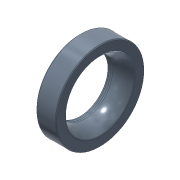
# Autodesk Inventor part: NA-45-h-Crown-129
Saved by Autodesk Inventor 2020.2 (Build 242310000, 310)
## iProperties
Created: 2020-09-21
Part Number: NA-45-h-Crown-129
Material: 19 436.4
Description: STAHOVACI KROUZEK
Document SubType Name: Modeling
Designer: Jurek
Density: 7.85 g/cm^3
Appearance: Ocelově modrá
Mass: 172.989 g
Surface Area: 71.9063 cm^2
Volume: 22.0368 cm^3
User Status: Rozpracováno
Category: B
Hmotnost (kg): 0,17
Rozmer_A: 60
Rozmer_B: 0
Rozmer_C: 0
Rozmer_D: 14
Rada vyrobku: 4100
Prumer nadobky: 45
Cislo artiklu: 4451101286
C. variantniho vykresu: NA-45-h-Crown-127
Jednotka: ks
Cisty rozmer: =Ø<Rozmer_A> - <Rozmer_D>
Predpona: Ø
Stroj na lince: Stahovací lis
RAZ Poznamka 1: ISO 2768-mH
RAZ Poznamka 2: NEOZNAČENÉ HRANY OJEHLIT
RAZ Poznamka 3: KALIT NA 58 - 60 HRc
DXF: Ne
QAD_code: M
Rizeni davek: L
Author: Správce
Revision Number: 00
Autodesk Inventor part; units mm, degrees
ref_plane "YZ Plane" through (0, 0, 0) normal (1, 0, 0) x (0, 1, 0)
ref_plane "XZ Plane" through (0, 0, 0) normal (0, 1, 0) x (-1, 0, 0)
ref_plane "XY Plane" through (0, 0, 0) normal (0, 0, 1) x (1, 0, 0)
sketch "Náčrt1" plane through (0, 0, 0) normal (0, 0, 1) x (1, 0, 0)
  line L0 (0, 0) -> (14.198, 0)
  line L1 (0, 19.135) -> (0, 30)
  line L2 (0, 30) -> (14, 30)
  line L3 (14, 30) -> (14, 23.8859)
  line L4 (3.5, 18.76) -> (2.3, 18.76)
  arc A0 (3.5, 18.76) -> (13.7308, 23.2033) centre (3.5, 32.76) ccw
  arc A1 (13.7308, 23.2033) -> (14, 23.8859) centre (13, 23.8859) ccw
  line L5 (0.3, 18.835) -> (1.0738, 18.835)
  line L6 (1.0738, 18.835) -> (2.3, 18.76)
  arc A2 (0, 19.135) -> (0.3, 18.835) centre (0.3, 19.135) ccw
  point P0 (0, 18.835)
  dimension "d0" = 60
  dimension "d1" = 37.52
  dimension "d4" = 14
  dimension "d18" = 1
  dimension "d21" = 14
  dimension "d25" = 10.5
  dimension "d26" = 1.2
  dimension "d27" = 37.67
  dimension "d28" = 3.5
  dimension "d29" = 0.3
  dimension "d32" = 5.1259
  constraints: 14 end point, 6 point on circle, 5 tangent, 3 centre point, 3 point on line, 2 parallel, 2 perpendicular, 1 horizontal
  measures "d0" diameter of L2 L0
  measures "d1" diameter of L4 L0
  measures "d4" distance between parallel lines of L3 L1
  measures "d18" radius of A1
  measures "d21" radius of A0
  measures "d25" distance from line of L4.start L3
  measures "d26" distance of L4.start L4.end
  measures "d27" diameter of L5 L0
  measures "d28" angle of L6 L4
  measures "d29" radius of A2
  measures "d32" distance from line of L3.end L4
revolve "Rotace1" add sketch "Náčrt1" angle 360 about axis through (0, 0, 0) along (1, 0, 0)
chamfer "Zkosení1" distance 1 angle 45 1 edges at (0, -30, 0)
chamfer "Zkosení2" distance 0.5 angle 45 1 edges at (14, -30, 0)
equation "\"Rozmer_B\" = 0"
equation "\"Rozmer_C\" = 0"
equation "\"Rozmer_D\" = d21"
